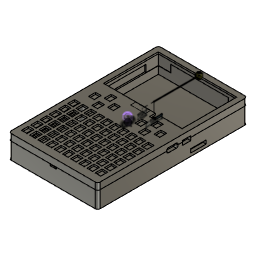
EPI (Autodesk Fusion 360 design; units mm, degrees)
Autodesk Fusion 360 part; units mm, degrees
(part 1 of 2)
sketch "Esquisse1" plane through (0, 0, 0) normal (0, 0, 1) x (1, 0, 0)
  line L0 (33.05, -57.68) -> (-33.05, -57.68)
  line L1 (-33.05, -57.68) -> (-33.05, 57.68)
  line L2 (-33.05, 57.68) -> (33.05, 57.68)
  line L3 (33.05, 57.68) -> (33.05, -57.68)
  line L4 (33.05, -57.68) -> (-33.05, 57.68) construction
  line L5 (-33.05, -57.68) -> (33.05, 57.68) construction
  line L6 (0, 57.68) -> (0, -57.68) construction
  line L7 (31.85, 12.08) -> (-31.85, 12.08)
  line L8 (-31.85, 12.08) -> (-31.85, 56.38)
  line L9 (-31.85, 56.38) -> (31.85, 56.38)
  line L10 (31.85, 56.38) -> (31.85, 12.08)
  line L11 (31.85, 12.08) -> (-31.85, 56.38) construction
  line L12 (-31.85, 12.08) -> (31.85, 56.38) construction
  line L13 (0, -57.68) -> (0, -51.48) construction
  line L14 (0, -51.48) -> (-3.325, -51.48) construction
  line L15 (-1.075, -48.68) -> (-5.575, -48.68)
  line L16 (-5.575, -48.68) -> (-5.575, -54.28)
  line L17 (-5.575, -54.28) -> (-1.075, -54.28)
  line L18 (-1.075, -54.28) -> (-1.075, -48.68)
  line L19 (-1.075, -48.68) -> (-5.575, -54.28) construction
  line L20 (-5.575, -48.68) -> (-1.075, -54.28) construction
  line L21 (-27.675, -48.68) -> (-32.175, -48.68)
  line L22 (-32.175, -48.68) -> (-32.175, -54.28)
  line L23 (-32.175, -54.28) -> (-27.675, -54.28)
  line L24 (-27.675, -54.28) -> (-27.675, -48.68)
  line L25 (-21.025, -48.68) -> (-25.525, -48.68)
  line L26 (-25.525, -48.68) -> (-25.525, -54.28)
  line L27 (-25.525, -54.28) -> (-21.025, -54.28)
  line L28 (-21.025, -54.28) -> (-21.025, -48.68)
  line L29 (-14.375, -48.68) -> (-18.875, -48.68)
  line L30 (-18.875, -48.68) -> (-18.875, -54.28)
  line L31 (-18.875, -54.28) -> (-14.375, -54.28)
  line L32 (-14.375, -54.28) -> (-14.375, -48.68)
  line L33 (-7.725, -48.68) -> (-12.225, -48.68)
  line L34 (-12.225, -48.68) -> (-12.225, -54.28)
  line L35 (-12.225, -54.28) -> (-7.725, -54.28)
  line L36 (-7.725, -54.28) -> (-7.725, -48.68)
  line L37 (5.575, -48.68) -> (1.075, -48.68)
  line L38 (1.075, -48.68) -> (1.075, -54.28)
  line L39 (1.075, -54.28) -> (5.575, -54.28)
  line L40 (5.575, -54.28) -> (5.575, -48.68)
  line L41 (12.225, -48.68) -> (7.725, -48.68)
  line L42 (7.725, -48.68) -> (7.725, -54.28)
  line L43 (7.725, -54.28) -> (12.225, -54.28)
  line L44 (12.225, -54.28) -> (12.225, -48.68)
  line L45 (18.875, -48.68) -> (14.375, -48.68)
  line L46 (14.375, -48.68) -> (14.375, -54.28)
  line L47 (14.375, -54.28) -> (18.875, -54.28)
  line L48 (18.875, -54.28) -> (18.875, -48.68)
  line L49 (25.525, -48.68) -> (21.025, -48.68)
  line L50 (21.025, -48.68) -> (21.025, -54.28)
  line L51 (21.025, -54.28) -> (25.525, -54.28)
  line L52 (25.525, -54.28) -> (25.525, -48.68)
  line L53 (32.175, -48.68) -> (27.675, -48.68)
  line L54 (27.675, -48.68) -> (27.675, -54.28)
  line L55 (27.675, -54.28) -> (32.175, -54.28)
  line L56 (32.175, -54.28) -> (32.175, -48.68)
  line L57 (-27.675, -41.17) -> (-32.175, -41.17)
  line L58 (-32.175, -41.17) -> (-32.175, -46.77)
  line L59 (-32.175, -46.77) -> (-27.675, -46.77)
  line L60 (-27.675, -46.77) -> (-27.675, -41.17)
  line L61 (-21.025, -41.17) -> (-25.525, -41.17)
  line L62 (-25.525, -41.17) -> (-25.525, -46.77)
  line L63 (-25.525, -46.77) -> (-21.025, -46.77)
  line L64 (-21.025, -46.77) -> (-21.025, -41.17)
  line L65 (-14.375, -41.17) -> (-18.875, -41.17)
  line L66 (-18.875, -41.17) -> (-18.875, -46.77)
  line L67 (-18.875, -46.77) -> (-14.375, -46.77)
  line L68 (-14.375, -46.77) -> (-14.375, -41.17)
  line L69 (-7.725, -41.17) -> (-12.225, -41.17)
  line L70 (-12.225, -41.17) -> (-12.225, -46.77)
  line L71 (-12.225, -46.77) -> (-7.725, -46.77)
  line L72 (-7.725, -46.77) -> (-7.725, -41.17)
  line L73 (-1.075, -41.17) -> (-5.575, -41.17)
  line L74 (-5.575, -41.17) -> (-5.575, -46.77)
  line L75 (-5.575, -46.77) -> (-1.075, -46.77)
  line L76 (-1.075, -46.77) -> (-1.075, -41.17)
  line L77 (5.575, -41.17) -> (1.075, -41.17)
  line L78 (1.075, -41.17) -> (1.075, -46.77)
  line L79 (1.075, -46.77) -> (5.575, -46.77)
  line L80 (5.575, -46.77) -> (5.575, -41.17)
  line L81 (12.225, -41.17) -> (7.725, -41.17)
  line L82 (7.725, -41.17) -> (7.725, -46.77)
  line L83 (7.725, -46.77) -> (12.225, -46.77)
  line L84 (12.225, -46.77) -> (12.225, -41.17)
  line L85 (18.875, -41.17) -> (14.375, -41.17)
  line L86 (14.375, -41.17) -> (14.375, -46.77)
  line L87 (14.375, -46.77) -> (18.875, -46.77)
  line L88 (18.875, -46.77) -> (18.875, -41.17)
  line L89 (25.525, -41.17) -> (21.025, -41.17)
  line L90 (21.025, -41.17) -> (21.025, -46.77)
  line L91 (21.025, -46.77) -> (25.525, -46.77)
  line L92 (25.525, -46.77) -> (25.525, -41.17)
  line L93 (32.175, -41.17) -> (27.675, -41.17)
  line L94 (27.675, -41.17) -> (27.675, -46.77)
  line L95 (27.675, -46.77) -> (32.175, -46.77)
  line L96 (32.175, -46.77) -> (32.175, -41.17)
  line L97 (-27.675, -33.66) -> (-32.175, -33.66)
  line L98 (-32.175, -33.66) -> (-32.175, -39.26)
  line L99 (-32.175, -39.26) -> (-27.675, -39.26)
  line L100 (-27.675, -39.26) -> (-27.675, -33.66)
  line L101 (-21.025, -33.66) -> (-25.525, -33.66)
  line L102 (-25.525, -33.66) -> (-25.525, -39.26)
  line L103 (-25.525, -39.26) -> (-21.025, -39.26)
  line L104 (-21.025, -39.26) -> (-21.025, -33.66)
  line L105 (-14.375, -33.66) -> (-18.875, -33.66)
  line L106 (-18.875, -33.66) -> (-18.875, -39.26)
  line L107 (-18.875, -39.26) -> (-14.375, -39.26)
  line L108 (-14.375, -39.26) -> (-14.375, -33.66)
  line L109 (-7.725, -33.66) -> (-12.225, -33.66)
  line L110 (-12.225, -33.66) -> (-12.225, -39.26)
  line L111 (-12.225, -39.26) -> (-7.725, -39.26)
  line L112 (-7.725, -39.26) -> (-7.725, -33.66)
  line L113 (-1.075, -33.66) -> (-5.575, -33.66)
  line L114 (-5.575, -33.66) -> (-5.575, -39.26)
  line L115 (-5.575, -39.26) -> (-1.075, -39.26)
  line L116 (-1.075, -39.26) -> (-1.075, -33.66)
  line L117 (5.575, -33.66) -> (1.075, -33.66)
  line L118 (1.075, -33.66) -> (1.075, -39.26)
  line L119 (1.075, -39.26) -> (5.575, -39.26)
  line L120 (5.575, -39.26) -> (5.575, -33.66)
  line L121 (12.225, -33.66) -> (7.725, -33.66)
  line L122 (7.725, -33.66) -> (7.725, -39.26)
  line L123 (7.725, -39.26) -> (12.225, -39.26)
  line L124 (12.225, -39.26) -> (12.225, -33.66)
  line L125 (18.875, -33.66) -> (14.375, -33.66)
  line L126 (14.375, -33.66) -> (14.375, -39.26)
  line L127 (14.375, -39.26) -> (18.875, -39.26)
  line L128 (18.875, -39.26) -> (18.875, -33.66)
  line L129 (25.525, -33.66) -> (21.025, -33.66)
  line L130 (21.025, -33.66) -> (21.025, -39.26)
  line L131 (21.025, -39.26) -> (25.525, -39.26)
  line L132 (25.525, -39.26) -> (25.525, -33.66)
  line L133 (32.175, -33.66) -> (27.675, -33.66)
  line L134 (27.675, -33.66) -> (27.675, -39.26)
  line L135 (27.675, -39.26) -> (32.175, -39.26)
  line L136 (32.175, -39.26) -> (32.175, -33.66)
  line L137 (-27.675, -26.15) -> (-32.175, -26.15)
  line L138 (-32.175, -26.15) -> (-32.175, -31.75)
  line L139 (-32.175, -31.75) -> (-27.675, -31.75)
  line L140 (-27.675, -31.75) -> (-27.675, -26.15)
  line L141 (-21.025, -26.15) -> (-25.525, -26.15)
  line L142 (-25.525, -26.15) -> (-25.525, -31.75)
  line L143 (-25.525, -31.75) -> (-21.025, -31.75)
  line L144 (-21.025, -31.75) -> (-21.025, -26.15)
  line L145 (-14.375, -26.15) -> (-18.875, -26.15)
  line L146 (-18.875, -26.15) -> (-18.875, -31.75)
  line L147 (-18.875, -31.75) -> (-14.375, -31.75)
  line L148 (-14.375, -31.75) -> (-14.375, -26.15)
  line L149 (-7.725, -26.15) -> (-12.225, -26.15)
  line L150 (-12.225, -26.15) -> (-12.225, -31.75)
  line L151 (-12.225, -31.75) -> (-7.725, -31.75)
  line L152 (-7.725, -31.75) -> (-7.725, -26.15)
  line L153 (-1.075, -26.15) -> (-5.575, -26.15)
  line L154 (-5.575, -26.15) -> (-5.575, -31.75)
  line L155 (-5.575, -31.75) -> (-1.075, -31.75)
  line L156 (-1.075, -31.75) -> (-1.075, -26.15)
  line L157 (5.575, -26.15) -> (1.075, -26.15)
  line L158 (1.075, -26.15) -> (1.075, -31.75)
  line L159 (1.075, -31.75) -> (5.575, -31.75)
  line L160 (5.575, -31.75) -> (5.575, -26.15)
  line L161 (12.225, -26.15) -> (7.725, -26.15)
  line L162 (7.725, -26.15) -> (7.725, -31.75)
  line L163 (7.725, -31.75) -> (12.225, -31.75)
  line L164 (12.225, -31.75) -> (12.225, -26.15)
  line L165 (18.875, -26.15) -> (14.375, -26.15)
  line L166 (14.375, -26.15) -> (14.375, -31.75)
  line L167 (14.375, -31.75) -> (18.875, -31.75)
  line L168 (18.875, -31.75) -> (18.875, -26.15)
  line L169 (25.525, -26.15) -> (21.025, -26.15)
  line L170 (21.025, -26.15) -> (21.025, -31.75)
  line L171 (21.025, -31.75) -> (25.525, -31.75)
  line L172 (25.525, -31.75) -> (25.525, -26.15)
  line L173 (32.175, -26.15) -> (27.675, -26.15)
  line L174 (27.675, -26.15) -> (27.675, -31.75)
  line L175 (27.675, -31.75) -> (32.175, -31.75)
  line L176 (32.175, -31.75) -> (32.175, -26.15)
  line L177 (-27.675, -18.64) -> (-32.175, -18.64)
  line L178 (-32.175, -18.64) -> (-32.175, -24.24)
  line L179 (-32.175, -24.24) -> (-27.675, -24.24)
  line L180 (-27.675, -24.24) -> (-27.675, -18.64)
  line L181 (-21.025, -18.64) -> (-25.525, -18.64)
  line L182 (-25.525, -18.64) -> (-25.525, -24.24)
  line L183 (-25.525, -24.24) -> (-21.025, -24.24)
  line L184 (-21.025, -24.24) -> (-21.025, -18.64)
  line L185 (-14.375, -18.64) -> (-18.875, -18.64)
  line L186 (-18.875, -18.64) -> (-18.875, -24.24)
  line L187 (-18.875, -24.24) -> (-14.375, -24.24)
  line L188 (-14.375, -24.24) -> (-14.375, -18.64)
  line L189 (-7.725, -18.64) -> (-12.225, -18.64)
  line L190 (-12.225, -18.64) -> (-12.225, -24.24)
  line L191 (-12.225, -24.24) -> (-7.725, -24.24)
  line L192 (-7.725, -24.24) -> (-7.725, -18.64)
  line L193 (-1.075, -18.64) -> (-5.575, -18.64)
  line L194 (-5.575, -18.64) -> (-5.575, -24.24)
  line L195 (-5.575, -24.24) -> (-1.075, -24.24)
  line L196 (-1.075, -24.24) -> (-1.075, -18.64)
  line L197 (5.575, -18.64) -> (1.075, -18.64)
  line L198 (1.075, -18.64) -> (1.075, -24.24)
  line L199 (1.075, -24.24) -> (5.575, -24.24)
  line L200 (5.575, -24.24) -> (5.575, -18.64)
  line L201 (12.225, -18.64) -> (7.725, -18.64)
  line L202 (7.725, -18.64) -> (7.725, -24.24)
  line L203 (7.725, -24.24) -> (12.225, -24.24)
  line L204 (12.225, -24.24) -> (12.225, -18.64)
  line L205 (18.875, -18.64) -> (14.375, -18.64)
  line L206 (14.375, -18.64) -> (14.375, -24.24)
  line L207 (14.375, -24.24) -> (18.875, -24.24)
  line L208 (18.875, -24.24) -> (18.875, -18.64)
  line L209 (25.525, -18.64) -> (21.025, -18.64)
  line L210 (21.025, -18.64) -> (21.025, -24.24)
  line L211 (21.025, -24.24) -> (25.525, -24.24)
  line L212 (25.525, -24.24) -> (25.525, -18.64)
  line L213 (32.175, -18.64) -> (27.675, -18.64)
  line L214 (27.675, -18.64) -> (27.675, -24.24)
  line L215 (27.675, -24.24) -> (32.175, -24.24)
  line L216 (32.175, -24.24) -> (32.175, -18.64)
  line L217 (-27.675, -11.13) -> (-32.175, -11.13)
  line L218 (-32.175, -11.13) -> (-32.175, -16.73)
  line L219 (-32.175, -16.73) -> (-27.675, -16.73)
  line L220 (-27.675, -16.73) -> (-27.675, -11.13)
  line L221 (-21.025, -11.13) -> (-25.525, -11.13)
  line L222 (-25.525, -11.13) -> (-25.525, -16.73)
  line L223 (-25.525, -16.73) -> (-21.025, -16.73)
  line L224 (-21.025, -16.73) -> (-21.025, -11.13)
  line L225 (-14.375, -11.13) -> (-18.875, -11.13)
  line L226 (-18.875, -11.13) -> (-18.875, -16.73)
  line L227 (-18.875, -16.73) -> (-14.375, -16.73)
  line L228 (-14.375, -16.73) -> (-14.375, -11.13)
  line L229 (-7.725, -11.13) -> (-12.225, -11.13)
  line L230 (-12.225, -11.13) -> (-12.225, -16.73)
  line L231 (-12.225, -16.73) -> (-7.725, -16.73)
  line L232 (-7.725, -16.73) -> (-7.725, -11.13)
  line L233 (-1.075, -11.13) -> (-5.575, -11.13)
  line L234 (-5.575, -11.13) -> (-5.575, -16.73)
  line L235 (-5.575, -16.73) -> (-1.075, -16.73)
  line L236 (-1.075, -16.73) -> (-1.075, -11.13)
  line L237 (5.575, -11.13) -> (1.075, -11.13)
  line L238 (1.075, -11.13) -> (1.075, -16.73)
  line L239 (1.075, -16.73) -> (5.575, -16.73)
  line L240 (5.575, -16.73) -> (5.575, -11.13)
  line L241 (12.225, -11.13) -> (7.725, -11.13)
  line L242 (7.725, -11.13) -> (7.725, -16.73)
  line L243 (7.725, -16.73) -> (12.225, -16.73)
  line L244 (12.225, -16.73) -> (12.225, -11.13)
  line L245 (18.875, -11.13) -> (14.375, -11.13)
  line L246 (14.375, -11.13) -> (14.375, -16.73)
  line L247 (14.375, -16.73) -> (18.875, -16.73)
  line L248 (18.875, -16.73) -> (18.875, -11.13)
  line L249 (25.525, -11.13) -> (21.025, -11.13)
  line L250 (21.025, -11.13) -> (21.025, -16.73)
  line L251 (21.025, -16.73) -> (25.525, -16.73)
  line L252 (25.525, -16.73) -> (25.525, -11.13)
  line L253 (32.175, -11.13) -> (27.675, -11.13)
  line L254 (27.675, -11.13) -> (27.675, -16.73)
  line L255 (27.675, -16.73) -> (32.175, -16.73)
  line L256 (32.175, -16.73) -> (32.175, -11.13)
  line L257 (-5.8196, -10.1565) -> (33.05, -10.1565)
  line L258 (33.05, 57.68) -> (33.05, -0.32) construction
  line L259 (33.05, -0.32) -> (26.57, -0.32) construction
  line L260 (26.57, -0.32) -> (11.1, -0.32) construction
  line L261 (13.35, -3.12) -> (8.85, -3.12)
  line L262 (8.85, -3.12) -> (8.85, 2.48)
  line L263 (8.85, 2.48) -> (13.35, 2.48)
  line L264 (13.35, 2.48) -> (13.35, -3.12)
  line L265 (13.35, -3.12) -> (8.85, 2.48) construction
  line L266 (8.85, -3.12) -> (13.35, 2.48) construction
  line L267 (28.82, -3.12) -> (24.32, -3.12)
  line L268 (24.32, -3.12) -> (24.32, 2.48)
  line L269 (24.32, 2.48) -> (28.82, 2.48)
  line L270 (28.82, 2.48) -> (28.82, -3.12)
  line L271 (28.82, -3.12) -> (24.32, 2.48) construction
  line L272 (24.32, -3.12) -> (28.82, 2.48) construction
  line L273 (18.835, -0.32) -> (18.835, 4.71) construction
  line L274 (18.835, -0.32) -> (18.835, -5.35) construction
  line L275 (21.085, 1.91) -> (16.585, 1.91)
  line L276 (16.585, 1.91) -> (16.585, 7.51)
  line L277 (16.585, 7.51) -> (21.085, 7.51)
  line L278 (21.085, 7.51) -> (21.085, 1.91)
  line L279 (21.085, 1.91) -> (16.585, 7.51) construction
  line L280 (16.585, 1.91) -> (21.085, 7.51) construction
  line L281 (21.085, -8.15) -> (16.585, -8.15)
  line L282 (16.585, -8.15) -> (16.585, -2.55)
  line L283 (16.585, -2.55) -> (21.085, -2.55)
  line L284 (21.085, -2.55) -> (21.085, -8.15)
  line L285 (21.085, -8.15) -> (16.585, -2.55) construction
  line L286 (16.585, -8.15) -> (21.085, -2.55) construction
  line L287 (-21.085, 1.91) -> (-16.585, 1.91)
  line L288 (-21.085, 7.51) -> (-21.085, 1.91)
  line L289 (-16.585, 7.51) -> (-21.085, 7.51)
  line L290 (-16.585, 1.91) -> (-16.585, 7.51)
  line L291 (-21.085, -2.55) -> (-21.085, -8.15)
  line L292 (-16.585, -2.55) -> (-21.085, -2.55)
  line L293 (-16.585, -8.15) -> (-16.585, -2.55)
  line L294 (-21.085, -8.15) -> (-16.585, -8.15)
  line L295 (-24.32, -3.12) -> (-24.32, 2.48)
  line L296 (-24.32, 2.48) -> (-28.82, 2.48)
  line L297 (-28.82, 2.48) -> (-28.82, -3.12)
  line L298 (-28.82, -3.12) -> (-24.32, -3.12)
  line L299 (-8.85, -3.12) -> (-8.85, 2.48)
  line L300 (-8.85, 2.48) -> (-13.35, 2.48)
  line L301 (-13.35, 2.48) -> (-13.35, -3.12)
  line L302 (-13.35, -3.12) -> (-8.85, -3.12)
  line L303 (33.05, 57.68) -> (33.05, 10.18) construction
  line L304 (33.05, 10.18) -> (12.35, 10.18) construction
  line L305 (14.6, 7.38) -> (10.1, 7.38)
  line L306 (10.1, 7.38) -> (10.1, 12.98)
  line L307 (10.1, 12.98) -> (14.6, 12.98)
  line L308 (14.6, 12.98) -> (14.6, 7.38)
  line L309 (14.6, 7.38) -> (10.1, 12.98) construction
  line L310 (10.1, 7.38) -> (14.6, 12.98) construction
  line L311 (0, 12.08) -> (6, 12.08)
  line L312 (6, 12.08) -> (6, 8.08)
  line L313 (6, 8.08) -> (0, 8.08)
  line L314 (0, 8.08) -> (0, 12.08)
  line L315 (0, 12.08) -> (-6, 12.08)
  line L316 (-6, 12.08) -> (-6, 8.08)
  line L317 (-6, 8.08) -> (0, 8.08)
  line L318 (0, 8.08) -> (0, 12.08)
  line L319 (33.45, 58.08) -> (33.45, -58.08)
  line L320 (33.45, -58.08) -> (-33.45, -58.08)
  line L321 (-33.45, -58.08) -> (-33.45, 58.08)
  line L322 (-33.45, 58.08) -> (33.45, 58.08)
  line L323 (36.05, 58.68) -> (36.05, -58.68)
  line L324 (34.05, -60.68) -> (-34.05, -60.68)
  line L325 (-36.05, -58.68) -> (-36.05, 58.68)
  line L326 (-34.05, 60.68) -> (34.05, 60.68)
  arc A0 (-34.05, 60.68) -> (-36.05, 58.68) centre (-34.05, 58.68) ccw
  arc A1 (36.05, 58.68) -> (34.05, 60.68) centre (34.05, 58.68) ccw
  arc A2 (34.05, -60.68) -> (36.05, -58.68) centre (34.05, -58.68) ccw
  arc A3 (-36.05, -58.68) -> (-34.05, -60.68) centre (-34.05, -58.68) ccw
  line L327 (33.45, 58.08) -> (23.45, 58.08)
  line L328 (33.45, 58.08) -> (33.45, 48.08)
  line L329 (33.45, 48.08) -> (34.45, 48.08)
  line L330 (23.45, 58.08) -> (23.45, 59.08)
  line L331 (34.45, 48.08) -> (34.45, 59.08)
  line L332 (23.45, 59.08) -> (34.45, 59.08)
  line L333 (33.45, -58.08) -> (23.45, -58.08)
  line L334 (33.45, -58.08) -> (33.45, -48.08)
  line L335 (33.45, -48.08) -> (34.45, -48.08)
  line L336 (23.45, -58.08) -> (23.45, -59.08)
  line L337 (34.45, -48.08) -> (34.45, -59.08)
  line L338 (23.45, -59.08) -> (34.45, -59.08)
  line L339 (34.65, -47.88) -> (34.65, -59.28)
  line L340 (23.25, -59.28) -> (34.65, -59.28)
  line L341 (23.25, -57.88) -> (23.25, -59.28)
  line L342 (33.25, -57.88) -> (23.25, -57.88)
  line L343 (33.25, -57.88) -> (33.25, -47.88)
  line L344 (33.25, -47.88) -> (34.65, -47.88)
  line L345 (23.25, 59.28) -> (34.65, 59.28)
  line L346 (34.65, 47.88) -> (34.65, 59.28)
  line L347 (33.25, 47.88) -> (34.65, 47.88)
  line L348 (33.25, 57.88) -> (33.25, 47.88)
  line L349 (33.25, 57.88) -> (23.25, 57.88)
  line L350 (23.25, 57.88) -> (23.25, 59.28)
  line L351 (-34.45, 48.08) -> (-34.45, 59.08)
  line L352 (-23.45, 59.08) -> (-34.45, 59.08)
  line L353 (-23.25, 59.28) -> (-34.65, 59.28)
  line L354 (-34.65, 47.88) -> (-34.65, 59.28)
  line L355 (-33.25, 47.88) -> (-34.65, 47.88)
  line L356 (-33.45, 48.08) -> (-34.45, 48.08)
  line L357 (-23.25, 57.88) -> (-23.25, 59.28)
  line L358 (-23.45, 58.08) -> (-23.45, 59.08)
  line L359 (-34.45, -48.08) -> (-34.45, -59.08)
  line L360 (-34.65, -47.88) -> (-34.65, -59.28)
  line L361 (-33.25, -47.88) -> (-34.65, -47.88)
  line L362 (-33.45, -48.08) -> (-34.45, -48.08)
  line L363 (-23.25, -59.28) -> (-34.65, -59.28)
  line L364 (-23.45, -59.08) -> (-34.45, -59.08)
  line L365 (-23.25, -57.88) -> (-23.25, -59.28)
  line L366 (-23.45, -58.08) -> (-23.45, -59.08)
  line L367 (-34.65, -47.88) -> (-34.65, 47.88)
  point P0 (0, 34.23)
  point P1 (-3.325, -51.48)
  point P2 (11.1, -0.32)
  point P3 (26.57, -0.32)
  point P4 (18.835, 4.71)
  point P5 (18.835, -5.35)
  point P6 (12.35, 10.18)
  dimension "d12" = 66.1
  dimension "d13" = 115.36
  dimension "d14" = 63.7
  dimension "d15" = 44.3
  dimension "d16" = 1.3
  dimension "d20" = 6.2
  dimension "d21" = 3.325
  dimension "d22" = 4.5
  dimension "d23" = 5.6
  dimension "d26" = 6.65
  dimension "d27" = 7.51
  dimension "d33" = 58
  dimension "d34" = 6.48
  dimension "d35" = 15.47
  dimension "d36" = 4.5
  dimension "d37" = 5.6
  dimension "d38" = 4.5
  dimension "d39" = 5.6
  dimension "d40" = 5.03
  dimension "d41" = 5.03
  dimension "d42" = 4.5
  dimension "d43" = 5.6
  dimension "d44" = 4.5
  dimension "d45" = 5.6
  dimension "d46" = 47.5
  dimension "d47" = 20.7
  dimension "d48" = 4.5
  dimension "d49" = 5.6
  dimension "d74" = 6
  dimension "d75" = 4
  dimension "d76" = 6
  dimension "d77" = 4
  dimension "d83" = 2
  dimension "d98" = 10
  dimension "d99" = 10
  dimension "d101" = 1
  dimension "d102" = 1
  dimension "d103" = 11
  dimension "d104" = 11
  dimension "d106" = 10
  dimension "d107" = 10
  dimension "d108" = 1
  dimension "d109" = 1
  dimension "d110" = 11
  dimension "d111" = 11
  constraint horizontal L0
  constraint perpendicular L0 L1
  constraint parallel L0 L2
  constraint parallel L1 L3
  constraint coincident L4 origin
  constraint coincident L5 origin
  constraint midpoint L2 L6.start
  constraint midpoint L0 L6.end
  constraint horizontal L7
  constraint perpendicular L7 L8
  constraint parallel L7 L9
  constraint parallel L8 L10
  constraint coincident L11 P0
  constraint coincident L12 P0
  constraint coincident L6 P0
  constraint perpendicular L0 L13
  constraint perpendicular L3 L14
  constraint horizontal L15
  constraint perpendicular L15 L16
  constraint parallel L15 L17
  constraint parallel L16 L18
  constraint coincident L19 P1
  constraint coincident L20 P1
  constraint coincident P1 L14.end
  constraint coincident L3 L257.end
  constraint perpendicular L3 L257
  constraint perpendicular L7 L258
  constraint perpendicular L258 L259
  constraint perpendicular L6 L260
  constraint horizontal L261
  constraint perpendicular L261 L262
  constraint parallel L261 L263
  constraint parallel L262 L264
  constraint coincident L265 P2
  constraint coincident L266 P2
  constraint coincident P2 L260.end
  constraint horizontal L267
  constraint perpendicular L267 L268
  constraint parallel L267 L269
  constraint parallel L268 L270
  constraint coincident L271 P3
  constraint coincident L272 P3
  constraint coincident P3 L259.end
  constraint midpoint L260 L273.start
  constraint perpendicular L7 L273
  constraint perpendicular L260 L274
  constraint horizontal L275
  constraint perpendicular L275 L276
  constraint parallel L275 L277
  constraint parallel L276 L278
  constraint coincident L279 P4
  constraint coincident L280 P4
  constraint coincident P4 L273.end
  constraint horizontal L281
  constraint perpendicular L281 L282
  constraint parallel L281 L283
  constraint parallel L282 L284
  constraint coincident L285 P5
  constraint coincident L286 P5
  constraint coincident P5 L274.end
  constraint symmetric L6 L261.start L301.end
  constraint symmetric L6 L261.end L299.start
  constraint symmetric L6 L262.end L299.end
  constraint symmetric L6 L263.end L300.end
  constraint symmetric L6 L267.start L297.end
  constraint symmetric L6 L267.end L295.start
  constraint symmetric L6 L268.end L295.end
  constraint symmetric L6 L269.end L296.end
  constraint symmetric L6 L275.start L287.start
  constraint symmetric L6 L275.end L287.end
  constraint symmetric L6 L276.end L289.start
  constraint symmetric L6 L277.end L288.start
  constraint symmetric L6 L281.start L291.end
  constraint symmetric L6 L281.end L293.start
  constraint symmetric L6 L282.end L292.start
  constraint symmetric L6 L283.end L291.start
  constraint perpendicular L2 L303
  constraint perpendicular L303 L304
  constraint horizontal L305
  constraint perpendicular L305 L306
  constraint parallel L305 L307
  constraint parallel L306 L308
  constraint coincident L309 P6
  constraint coincident L310 P6
  constraint coincident P6 L304.end
  constraint coincident L5 L257.start
  constraint horizontal L311
  constraint vertical L312
  constraint horizontal L313
  constraint vertical L314
  constraint midpoint L7 L311.start
  constraint horizontal L315
  constraint vertical L316
  constraint horizontal L317
  constraint vertical L318
  constraint tangent L325 A0
  constraint tangent L326 A0
  constraint tangent L323 A1
  constraint tangent L326 A1
  constraint equal A0 A1
  constraint tangent L323 A2
  constraint tangent L324 A2
  constraint equal A0 A2
  constraint tangent L324 A3
  constraint tangent L325 A3
  constraint equal A0 A3
  constraint coincident L322 L327.end
  constraint coincident L319 L328.end
  constraint perpendicular L328 L329
  constraint perpendicular L327 L330
  constraint perpendicular L329 L331
  constraint perpendicular L330 L332
  constraint perpendicular L319 L333
  constraint perpendicular L320 L334
  constraint perpendicular L334 L335
  constraint perpendicular L333 L336
  constraint perpendicular L335 L337
  constraint perpendicular L336 L338
  constraint symmetric L6 L327.end L358.start
  constraint symmetric L6 L328.end L356.start
  constraint symmetric L6 L329.end L351.start
  constraint symmetric L6 L330.end L352.start
  constraint symmetric L6 L331.end L351.end
  constraint symmetric L6 L333.end L366.start
  constraint symmetric L6 L334.end L362.start
  constraint symmetric L6 L335.end L359.start
  constraint symmetric L6 L336.end L364.start
  constraint symmetric L6 L337.end L359.end
  constraint symmetric L6 L339.start L360.start
  constraint symmetric L6 L339.end L360.end
  constraint symmetric L6 L340.start L363.start
  constraint symmetric L6 L341.start L365.start
  constraint symmetric L6 L343.end L361.start
  constraint symmetric L6 L345.start L353.start
  constraint symmetric L6 L345.end L353.end
  constraint symmetric L6 L346.start L354.start
  constraint symmetric L6 L347.start L355.start
  constraint symmetric L6 L349.end L357.start
  measures "d12" distance of L1.end L2.end
  measures "d13" distance of L0.end L1.end
  measures "d14" distance of L8.end L9.end
  measures "d15" distance of L7.end L8.end
  measures "d16" distance of L2 L9
  measures "d20" distance of L6.end L13.end
  measures "d21" distance of L13.end P1
  measures "d22" distance of L16.end L17.end
  measures "d23" distance of L15.end L16.end
  measures "d33" distance of L2.end L258.end
  measures "d34" distance of L258.end P3
  measures "d35" distance of P3 P2
  measures "d36" distance of L262.end L263.end
  measures "d37" distance of L261.end L262.end
  measures "d38" distance of L268.end L269.end
  measures "d39" distance of L267.end L268.end
  measures "d40" distance of L273.start P4
  measures "d41" distance of L273.start P5
  measures "d42" distance of L276.end L277.end
  measures "d43" distance of L275.end L276.end
  measures "d44" distance of L282.end L283.end
  measures "d45" distance of L281.end L282.end
  measures "d46" distance of L2.end L303.end
  measures "d47" distance of L303.end P6
  measures "d48" distance of L306.end L307.end
  measures "d49" distance of L305.end L306.end
  measures "d74" distance of L311.start L311.end
  measures "d75" distance of L311.start L313.end
  measures "d76" distance of L311.start L315.end
  measures "d77" distance of L311.start L313.end
  measures "d83" radius of A0
  measures "d98" distance of L319.start L327.end
  measures "d99" distance of L319.start L328.end
  measures "d101" distance of L328.end L329.end
  measures "d102" distance of L327.end L330.end
  measures "d103" distance of L329.end L331.end
  measures "d104" distance of L330.end L331.end
  measures "d106" distance of L319.end L333.end
  measures "d107" distance of L319.end L334.end
  measures "d108" distance of L334.end L335.end
  measures "d109" distance of L333.end L336.end
  measures "d110" distance of L335.end L337.end
  measures "d111" distance of L336.end L337.end
sketch "Esquisse2" plane through (0, 0, 0) normal (1, 0, 0) x (0, 1, 0)
  line L0 (0, 0) -> (0, -4) construction
  line L1 (3.15, -2.2) -> (-3.15, -2.2)
  line L2 (-4.65, -3.7) -> (-4.65, -4.3)
  line L3 (-3.15, -5.8) -> (3.15, -5.8)
  line L4 (4.65, -4.3) -> (4.65, -3.7)
  line L5 (4.65, -2.2) -> (-4.65, -5.8) construction
  line L6 (-4.65, -2.2) -> (4.65, -5.8) construction
  arc A0 (-3.15, -2.2) -> (-4.65, -3.7) centre (-3.15, -3.7) ccw
  arc A1 (-4.65, -4.3) -> (-3.15, -5.8) centre (-3.15, -4.3) ccw
  arc A2 (4.65, -3.7) -> (3.15, -2.2) centre (3.15, -3.7) ccw
  arc A3 (3.15, -5.8) -> (4.65, -4.3) centre (3.15, -4.3) ccw
  line L7 (57.68, 0) -> (11.56, 0) construction
  line L8 (11.56, 0) -> (11.56, -4.58) construction
  line L9 (14.91, -2.83) -> (8.21, -2.83)
  line L10 (8.21, -2.83) -> (8.21, -6.33)
  line L11 (8.21, -6.33) -> (14.91, -6.33)
  line L12 (14.91, -6.33) -> (14.91, -2.83)
  line L13 (14.91, -2.83) -> (8.21, -6.33) construction
  line L14 (8.21, -2.83) -> (14.91, -6.33) construction
  line L15 (57.68, 0) -> (21.08, 0)
  line L16 (21.08, 0) -> (21.08, -13.5) construction
  line L17 (27.38, -15) -> (14.78, -15)
  line L18 (14.78, -15) -> (14.78, -12)
  line L19 (14.78, -12) -> (27.38, -12)
  line L20 (27.38, -12) -> (27.38, -15)
  line L21 (27.38, -15) -> (14.78, -12) construction
  line L22 (14.78, -15) -> (27.38, -12) construction
  point P0 (-0.32, 0)
  point P1 (0, -4)
  point P2 (57.68, 0)
  point P3 (11.56, -4.58)
  point P4 (21.08, -13.5)
  dimension "d60" = 4
  dimension "d63" = 9.3
  dimension "d64" = 3.6
  dimension "d65" = 1.5
  dimension "d66" = 46.12
  dimension "d67" = 4.58
  dimension "d70" = 6.7
  dimension "d71" = 3.5
  dimension "d130" = 36.6
  dimension "d131" = 13.5
  dimension "d132" = 12.6
  dimension "d133" = 3
  constraint coincident L0.start origin
  constraint vertical L0
  constraint horizontal L1
  constraint perpendicular L1 L2
  constraint parallel L1 L3
  constraint parallel L2 L4
  constraint coincident L5 P1
  constraint coincident L6 P1
  constraint coincident P1 L0.end
  constraint coincident L6.start L2
  constraint coincident L6.start L1
  constraint tangent L2 A0
  constraint tangent L1 A0
  constraint coincident L5.end L3
  constraint coincident L5.end L2
  constraint tangent L3 A1
  constraint tangent L2 A1
  constraint equal A0 A1
  constraint coincident L5.start L1
  constraint coincident L5.start L4
  constraint tangent L1 A2
  constraint tangent L4 A2
  constraint equal A0 A2
  constraint coincident L6.end L3
  constraint coincident L6.end L4
  constraint tangent L3 A3
  constraint tangent L4 A3
  constraint equal A0 A3
  constraint coincident P2 L7.start
  constraint horizontal L7
  constraint perpendicular L3 L8
  constraint horizontal L9
  constraint perpendicular L9 L10
  constraint parallel L9 L11
  constraint parallel L10 L12
  constraint coincident L13 P3
  constraint coincident L14 P3
  constraint coincident P3 L8.end
  constraint parallel L7 L15
  constraint perpendicular L15 L16
  constraint horizontal L17
  constraint perpendicular L17 L18
  constraint parallel L17 L19
  constraint parallel L18 L20
  constraint coincident L21 P4
  constraint coincident L22 P4
  constraint coincident P4 L16.end
  measures "d60" distance of L0.start P1
  measures "d63" distance of L5.end L6.end
  measures "d64" distance of L6.start L5.end
  measures "d65" radius of A0
  measures "d66" distance of P2 L7.end
  measures "d67" distance of L7.end P3
  measures "d70" distance of L10.end L11.end
  measures "d71" distance of L9.end L10.end
  measures "d130" distance of P2 L15.end
  measures "d131" distance of L15.end P4
  measures "d132" distance of L18.end L19.end
  measures "d133" distance of L17.end L18.end
extrude "Extrusion7" add sketch "Esquisse1" along normal blind 1.4 contours L0 L1 L2 L3 | L7 L311 L312 L313 L314 L318 | L7 L314 L315 L316 L317 L318 | L319 L322 L327 L328 L329 L330 L331 L332 | L319 L322 L327 L328 L347 L348 L349 L350 | L319 L322 L329 L330 L331 L332 L345 L346 L347 L350 | L319 L320 L321 L322 L341 L342 L343 L344 L347 L348 L349 L350 | L319 L320 L335 L336 L337 L338 L339 L340 L341 L344 | L319 L320 L333 L334 L341 L342 L343 L344 | L321 L322 L351 L352 L353 L354 L355 L356 L357 L358 | L319 L320 L333 L334 L335 L336 L337 L338 | L321 L322 L351 L352 L356 L358 | L321 L355 L361 L367 | L320 L321 L359 L360 L361 L362 L363 L364 L365 L366 | L320 L321 L359 L362 L364 L366 | L323 L324 L325 L326 A0 A1 A2 A3 makes body 1
extrude "Extrusion8" add sketch "Esquisse1" against normal blind 4 contours L319 L322 L327 L328 L329 L330 L331 L332 | L319 L322 L329 L330 L331 L332 L345 L346 L347 L350 | L319 L320 L335 L336 L337 L338 L339 L340 L341 L344 | L321 L322 L351 L352 L353 L354 L355 L356 L357 L358 | L319 L320 L333 L334 L335 L336 L337 L338 | L321 L322 L351 L352 L356 L358 | L321 L355 L361 L367 | L320 L321 L359 L360 L361 L362 L363 L364 L365 L366 | L320 L321 L359 L362 L364 L366 | L323 L324 L325 L326 A0 A1 A2 A3 bodies 1
extrude "Extrusion9" cut sketch "Esquisse1" along normal blind 1 contours L7 L311 L312 L313 L314 L318 | L7 L314 L315 L316 L317 L318 bodies 1
ref_plane "Plan de construction1" through (0, 0, -16) normal (0, 0, 1) x (1, 0, 0)
sketch "Esquisse3" plane through (0, 0, -16) normal (0, 0, 1) x (1, 0, 0)
  line L0 (-33.45, 58.08) -> (-33.45, -58.08)
  line L1 (-33.45, -58.08) -> (33.45, -58.08)
  line L2 (33.45, -58.08) -> (33.45, 58.08)
  line L3 (33.45, 58.08) -> (-33.45, 58.08)
  arc A0 (-34.05, 60.68) -> (-36.05, 58.68) centre (-33.45, 58.08) ccw
  line L4 (-34.05, 60.68) -> (34.05, 60.68)
  arc A1 (36.05, 58.68) -> (34.05, 60.68) centre (33.45, 58.08) ccw
  line L5 (36.05, 58.68) -> (36.05, -58.68)
  arc A2 (34.05, -60.68) -> (36.05, -58.68) centre (33.45, -58.08) ccw
  line L6 (34.05, -60.68) -> (-34.05, -60.68)
  arc A3 (-36.05, -58.68) -> (-34.05, -60.68) centre (-33.45, -58.08) ccw
  line L7 (-36.05, -58.68) -> (-36.05, 58.68)
  line L8 (5.575, -11.13) -> (5.575, -16.73)
  line L9 (5.575, -16.73) -> (1.075, -16.73)
  line L10 (1.075, -16.73) -> (1.075, -11.13)
  line L11 (1.075, -11.13) -> (5.575, -11.13)
  line L12 (18.875, -18.64) -> (18.875, -24.24)
  line L13 (18.875, -24.24) -> (14.375, -24.24)
  line L14 (14.375, -24.24) -> (14.375, -18.64)
  line L15 (14.375, -18.64) -> (18.875, -18.64)
  line L16 (5.575, -18.64) -> (5.575, -24.24)
  line L17 (5.575, -24.24) -> (1.075, -24.24)
  line L18 (1.075, -24.24) -> (1.075, -18.64)
  line L19 (1.075, -18.64) -> (5.575, -18.64)
  line L20 (-1.075, -18.64) -> (-1.075, -24.24)
  line L21 (-1.075, -24.24) -> (-5.575, -24.24)
  line L22 (-5.575, -24.24) -> (-5.575, -18.64)
  line L23 (-5.575, -18.64) -> (-1.075, -18.64)
  line L24 (-7.725, -18.64) -> (-7.725, -24.24)
  line L25 (-7.725, -24.24) -> (-12.225, -24.24)
  line L26 (-12.225, -24.24) -> (-12.225, -18.64)
  line L27 (-12.225, -18.64) -> (-7.725, -18.64)
  line L28 (-14.375, -18.64) -> (-14.375, -24.24)
  line L29 (-14.375, -24.24) -> (-18.875, -24.24)
  line L30 (-18.875, -24.24) -> (-18.875, -18.64)
  line L31 (-18.875, -18.64) -> (-14.375, -18.64)
  line L32 (-21.025, -18.64) -> (-21.025, -24.24)
  line L33 (-21.025, -24.24) -> (-25.525, -24.24)
  line L34 (-25.525, -24.24) -> (-25.525, -18.64)
  line L35 (-25.525, -18.64) -> (-21.025, -18.64)
  line L36 (-27.675, -18.64) -> (-27.675, -24.24)
  line L37 (-27.675, -24.24) -> (-32.175, -24.24)
  line L38 (-32.175, -24.24) -> (-32.175, -18.64)
  line L39 (-32.175, -18.64) -> (-27.675, -18.64)
  line L40 (32.175, -26.15) -> (32.175, -31.75)
  line L41 (32.175, -31.75) -> (27.675, -31.75)
  line L42 (27.675, -31.75) -> (27.675, -26.15)
  line L43 (27.675, -26.15) -> (32.175, -26.15)
  line L44 (25.525, -26.15) -> (25.525, -31.75)
  line L45 (25.525, -31.75) -> (21.025, -31.75)
  line L46 (21.025, -31.75) -> (21.025, -26.15)
  line L47 (21.025, -26.15) -> (25.525, -26.15)
  line L48 (18.875, -26.15) -> (18.875, -31.75)
  line L49 (18.875, -31.75) -> (14.375, -31.75)
  line L50 (14.375, -31.75) -> (14.375, -26.15)
  line L51 (14.375, -26.15) -> (18.875, -26.15)
  line L52 (12.225, -26.15) -> (12.225, -31.75)
  line L53 (12.225, -31.75) -> (7.725, -31.75)
  line L54 (7.725, -31.75) -> (7.725, -26.15)
  line L55 (7.725, -26.15) -> (12.225, -26.15)
  line L56 (5.575, -26.15) -> (5.575, -31.75)
  line L57 (5.575, -31.75) -> (1.075, -31.75)
  line L58 (1.075, -31.75) -> (1.075, -26.15)
  line L59 (1.075, -26.15) -> (5.575, -26.15)
  line L60 (-1.075, -26.15) -> (-1.075, -31.75)
  line L61 (-1.075, -31.75) -> (-5.575, -31.75)
  line L62 (-5.575, -31.75) -> (-5.575, -26.15)
  line L63 (-5.575, -26.15) -> (-1.075, -26.15)
  line L64 (-7.725, -26.15) -> (-7.725, -31.75)
  line L65 (-7.725, -31.75) -> (-12.225, -31.75)
  line L66 (-12.225, -31.75) -> (-12.225, -26.15)
  line L67 (-12.225, -26.15) -> (-7.725, -26.15)
  line L68 (-14.375, -26.15) -> (-14.375, -31.75)
  line L69 (-14.375, -31.75) -> (-18.875, -31.75)
  line L70 (-18.875, -31.75) -> (-18.875, -26.15)
  line L71 (-18.875, -26.15) -> (-14.375, -26.15)
  line L72 (-21.025, -26.15) -> (-21.025, -31.75)
  line L73 (-21.025, -31.75) -> (-25.525, -31.75)
  line L74 (-25.525, -31.75) -> (-25.525, -26.15)
  line L75 (-25.525, -26.15) -> (-21.025, -26.15)
  line L76 (-27.675, -26.15) -> (-27.675, -31.75)
  line L77 (-27.675, -31.75) -> (-32.175, -31.75)
  line L78 (-32.175, -31.75) -> (-32.175, -26.15)
  line L79 (-32.175, -26.15) -> (-27.675, -26.15)
  line L80 (25.525, -33.66) -> (25.525, -39.26)
  line L81 (25.525, -39.26) -> (21.025, -39.26)
  line L82 (21.025, -39.26) -> (21.025, -33.66)
  line L83 (21.025, -33.66) -> (25.525, -33.66)
  line L84 (32.175, -33.66) -> (32.175, -39.26)
  line L85 (32.175, -39.26) -> (27.675, -39.26)
  line L86 (27.675, -39.26) -> (27.675, -33.66)
  line L87 (27.675, -33.66) -> (32.175, -33.66)
  line L88 (18.875, -33.66) -> (18.875, -39.26)
  line L89 (18.875, -39.26) -> (14.375, -39.26)
  line L90 (14.375, -39.26) -> (14.375, -33.66)
  line L91 (14.375, -33.66) -> (18.875, -33.66)
  line L92 (12.225, -33.66) -> (12.225, -39.26)
  line L93 (12.225, -39.26) -> (7.725, -39.26)
  line L94 (7.725, -39.26) -> (7.725, -33.66)
  line L95 (7.725, -33.66) -> (12.225, -33.66)
  line L96 (5.575, -33.66) -> (5.575, -39.26)
  line L97 (5.575, -39.26) -> (1.075, -39.26)
  line L98 (1.075, -39.26) -> (1.075, -33.66)
  line L99 (1.075, -33.66) -> (5.575, -33.66)
  line L100 (-7.725, -33.66) -> (-7.725, -39.26)
  line L101 (-7.725, -39.26) -> (-12.225, -39.26)
  line L102 (-12.225, -39.26) -> (-12.225, -33.66)
  line L103 (-12.225, -33.66) -> (-7.725, -33.66)
  line L104 (-1.075, -33.66) -> (-1.075, -39.26)
  line L105 (-1.075, -39.26) -> (-5.575, -39.26)
  line L106 (-5.575, -39.26) -> (-5.575, -33.66)
  line L107 (-5.575, -33.66) -> (-1.075, -33.66)
  line L108 (-14.375, -33.66) -> (-14.375, -39.26)
  line L109 (-14.375, -39.26) -> (-18.875, -39.26)
  line L110 (-18.875, -39.26) -> (-18.875, -33.66)
  line L111 (-18.875, -33.66) -> (-14.375, -33.66)
  line L112 (-21.025, -33.66) -> (-21.025, -39.26)
  line L113 (-21.025, -39.26) -> (-25.525, -39.26)
  line L114 (-25.525, -39.26) -> (-25.525, -33.66)
  line L115 (-25.525, -33.66) -> (-21.025, -33.66)
  line L116 (-1.075, -41.17) -> (-1.075, -46.77)
  line L117 (-1.075, -46.77) -> (-5.575, -46.77)
  line L118 (-5.575, -46.77) -> (-5.575, -41.17)
  line L119 (-5.575, -41.17) -> (-1.075, -41.17)
  line L120 (5.575, -41.17) -> (5.575, -46.77)
  line L121 (5.575, -46.77) -> (1.075, -46.77)
  line L122 (1.075, -46.77) -> (1.075, -41.17)
  line L123 (1.075, -41.17) -> (5.575, -41.17)
  line L124 (12.225, -41.17) -> (12.225, -46.77)
  line L125 (12.225, -46.77) -> (7.725, -46.77)
  line L126 (7.725, -46.77) -> (7.725, -41.17)
  line L127 (7.725, -41.17) -> (12.225, -41.17)
  line L128 (18.875, -41.17) -> (18.875, -46.77)
  line L129 (18.875, -46.77) -> (14.375, -46.77)
  line L130 (14.375, -46.77) -> (14.375, -41.17)
  line L131 (14.375, -41.17) -> (18.875, -41.17)
  line L132 (25.525, -41.17) -> (25.525, -46.77)
  line L133 (25.525, -46.77) -> (21.025, -46.77)
  line L134 (21.025, -46.77) -> (21.025, -41.17)
  line L135 (21.025, -41.17) -> (25.525, -41.17)
  line L136 (-27.675, -33.66) -> (-27.675, -39.26)
  line L137 (-27.675, -39.26) -> (-32.175, -39.26)
  line L138 (-32.175, -39.26) -> (-32.175, -33.66)
  line L139 (-32.175, -33.66) -> (-27.675, -33.66)
  line L140 (32.175, -41.17) -> (32.175, -46.77)
  line L141 (32.175, -46.77) -> (27.675, -46.77)
  line L142 (27.675, -46.77) -> (27.675, -41.17)
  line L143 (27.675, -41.17) -> (32.175, -41.17)
  line L144 (12.225, -18.64) -> (12.225, -24.24)
  line L145 (12.225, -24.24) -> (7.725, -24.24)
  line L146 (7.725, -24.24) -> (7.725, -18.64)
  line L147 (7.725, -18.64) -> (12.225, -18.64)
  line L148 (25.525, -18.64) -> (25.525, -24.24)
  line L149 (25.525, -24.24) -> (21.025, -24.24)
  line L150 (21.025, -24.24) -> (21.025, -18.64)
  line L151 (21.025, -18.64) -> (25.525, -18.64)
  line L152 (32.175, -18.64) -> (32.175, -24.24)
  line L153 (32.175, -24.24) -> (27.675, -24.24)
  line L154 (27.675, -24.24) -> (27.675, -18.64)
  line L155 (27.675, -18.64) -> (32.175, -18.64)
  line L156 (-27.675, -11.13) -> (-27.675, -16.73)
  line L157 (-27.675, -16.73) -> (-32.175, -16.73)
  line L158 (-32.175, -16.73) -> (-32.175, -11.13)
  line L159 (-32.175, -11.13) -> (-27.675, -11.13)
  line L160 (-21.025, -11.13) -> (-21.025, -16.73)
  line L161 (-21.025, -16.73) -> (-25.525, -16.73)
  line L162 (-25.525, -16.73) -> (-25.525, -11.13)
  line L163 (-25.525, -11.13) -> (-21.025, -11.13)
  line L164 (-1.075, -11.13) -> (-1.075, -16.73)
  line L165 (-1.075, -16.73) -> (-5.575, -16.73)
  line L166 (-5.575, -16.73) -> (-5.575, -11.13)
  line L167 (-5.575, -11.13) -> (-1.075, -11.13)
  line L168 (-14.375, -11.13) -> (-14.375, -16.73)
  line L169 (-14.375, -16.73) -> (-18.875, -16.73)
  line L170 (-18.875, -16.73) -> (-18.875, -11.13)
  line L171 (-18.875, -11.13) -> (-14.375, -11.13)
  line L172 (-7.725, -11.13) -> (-7.725, -16.73)
  line L173 (-7.725, -16.73) -> (-12.225, -16.73)
  line L174 (-12.225, -16.73) -> (-12.225, -11.13)
  line L175 (-12.225, -11.13) -> (-7.725, -11.13)
  line L176 (5.575, -48.68) -> (5.575, -54.28)
  line L177 (5.575, -54.28) -> (1.075, -54.28)
  line L178 (1.075, -54.28) -> (1.075, -48.68)
  line L179 (1.075, -48.68) -> (5.575, -48.68)
  line L180 (-7.725, -48.68) -> (-7.725, -54.28)
  line L181 (-7.725, -54.28) -> (-12.225, -54.28)
  line L182 (-12.225, -54.28) -> (-12.225, -48.68)
  line L183 (-12.225, -48.68) -> (-7.725, -48.68)
  line L184 (-14.375, -48.68) -> (-14.375, -54.28)
  line L185 (-14.375, -54.28) -> (-18.875, -54.28)
  line L186 (-18.875, -54.28) -> (-18.875, -48.68)
  line L187 (-18.875, -48.68) -> (-14.375, -48.68)
  line L188 (-21.025, -48.68) -> (-21.025, -54.28)
  line L189 (-21.025, -54.28) -> (-25.525, -54.28)
  line L190 (-25.525, -54.28) -> (-25.525, -48.68)
  line L191 (-25.525, -48.68) -> (-21.025, -48.68)
  line L192 (-1.075, -48.68) -> (-1.075, -54.28)
  line L193 (-1.075, -54.28) -> (-5.575, -54.28)
  line L194 (-5.575, -54.28) -> (-5.575, -48.68)
  line L195 (-5.575, -48.68) -> (-1.075, -48.68)
  line L196 (-14.375, -41.17) -> (-14.375, -46.77)
  line L197 (-14.375, -46.77) -> (-18.875, -46.77)
  line L198 (-18.875, -46.77) -> (-18.875, -41.17)
  line L199 (-18.875, -41.17) -> (-14.375, -41.17)
  line L200 (-27.675, -48.68) -> (-27.675, -54.28)
  line L201 (-27.675, -54.28) -> (-32.175, -54.28)
  line L202 (-32.175, -54.28) -> (-32.175, -48.68)
  line L203 (-32.175, -48.68) -> (-27.675, -48.68)
  line L204 (10.1, 12.08) -> (-31.85, 12.08)
  line L205 (-31.85, 12.08) -> (-31.85, 56.38)
  line L206 (-31.85, 56.38) -> (31.85, 56.38)
  line L207 (31.85, 56.38) -> (31.85, 12.08)
  line L208 (31.85, 12.08) -> (14.6, 12.08)
  line L209 (14.6, 12.08) -> (14.6, 7.38)
  line L210 (14.6, 7.38) -> (10.1, 7.38)
  line L211 (10.1, 7.38) -> (10.1, 12.08)
  line L212 (12.225, -48.68) -> (12.225, -54.28)
  line L213 (12.225, -54.28) -> (7.725, -54.28)
  line L214 (7.725, -54.28) -> (7.725, -48.68)
  line L215 (7.725, -48.68) -> (12.225, -48.68)
  line L216 (18.875, -48.68) -> (18.875, -54.28)
  line L217 (18.875, -54.28) -> (14.375, -54.28)
  line L218 (14.375, -54.28) -> (14.375, -48.68)
  line L219 (14.375, -48.68) -> (18.875, -48.68)
  line L220 (25.525, -48.68) -> (25.525, -54.28)
  line L221 (25.525, -54.28) -> (21.025, -54.28)
  line L222 (21.025, -54.28) -> (21.025, -48.68)
  line L223 (21.025, -48.68) -> (25.525, -48.68)
  line L224 (32.175, -48.68) -> (32.175, -54.28)
  line L225 (32.175, -54.28) -> (27.675, -54.28)
  line L226 (27.675, -54.28) -> (27.675, -48.68)
  line L227 (27.675, -48.68) -> (32.175, -48.68)
  line L228 (-27.675, -41.17) -> (-27.675, -46.77)
  line L229 (-27.675, -46.77) -> (-32.175, -46.77)
  line L230 (-32.175, -46.77) -> (-32.175, -41.17)
  line L231 (-32.175, -41.17) -> (-27.675, -41.17)
  line L232 (-7.725, -41.17) -> (-7.725, -46.77)
  line L233 (-7.725, -46.77) -> (-12.225, -46.77)
  line L234 (-12.225, -46.77) -> (-12.225, -41.17)
  line L235 (-12.225, -41.17) -> (-7.725, -41.17)
  line L236 (-21.025, -41.17) -> (-21.025, -46.77)
  line L237 (-21.025, -46.77) -> (-25.525, -46.77)
  line L238 (-25.525, -46.77) -> (-25.525, -41.17)
  line L239 (-25.525, -41.17) -> (-21.025, -41.17)
  line L240 (-8.85, -3.12) -> (-13.35, -3.12)
  line L241 (-13.35, -3.12) -> (-13.35, 2.48)
  line L242 (-13.35, 2.48) -> (-8.85, 2.48)
  line L243 (-8.85, 2.48) -> (-8.85, -3.12)
  line L244 (-24.32, -3.12) -> (-28.82, -3.12)
  line L245 (-28.82, -3.12) -> (-28.82, 2.48)
  line L246 (-28.82, 2.48) -> (-24.32, 2.48)
  line L247 (-24.32, 2.48) -> (-24.32, -3.12)
  line L248 (-16.585, -8.15) -> (-21.085, -8.15)
  line L249 (-21.085, -8.15) -> (-21.085, -2.55)
  line L250 (-21.085, -2.55) -> (-16.585, -2.55)
  line L251 (-16.585, -2.55) -> (-16.585, -8.15)
  line L252 (16.585, -2.55) -> (21.085, -2.55)
  line L253 (21.085, -2.55) -> (21.085, -8.15)
  line L254 (21.085, -8.15) -> (16.585, -8.15)
  line L255 (16.585, -8.15) -> (16.585, -2.55)
  line L256 (-16.585, 7.51) -> (-16.585, 1.91)
  line L257 (-16.585, 1.91) -> (-21.085, 1.91)
  line L258 (-21.085, 1.91) -> (-21.085, 7.51)
  line L259 (-21.085, 7.51) -> (-16.585, 7.51)
  line L260 (16.585, 7.51) -> (21.085, 7.51)
  line L261 (21.085, 7.51) -> (21.085, 1.91)
  line L262 (21.085, 1.91) -> (16.585, 1.91)
  line L263 (16.585, 1.91) -> (16.585, 7.51)
  line L264 (24.32, 2.48) -> (28.82, 2.48)
  line L265 (28.82, 2.48) -> (28.82, -3.12)
  line L266 (28.82, -3.12) -> (24.32, -3.12)
  line L267 (24.32, -3.12) -> (24.32, 2.48)
  line L268 (8.85, 2.48) -> (13.35, 2.48)
  line L269 (13.35, 2.48) -> (13.35, -3.12)
  line L270 (13.35, -3.12) -> (8.85, -3.12)
  line L271 (8.85, -3.12) -> (8.85, 2.48)
  line L272 (32.175, -11.13) -> (32.175, -16.73)
  line L273 (32.175, -16.73) -> (27.675, -16.73)
  line L274 (27.675, -16.73) -> (27.675, -11.13)
  line L275 (27.675, -11.13) -> (32.175, -11.13)
  line L276 (25.525, -11.13) -> (25.525, -16.73)
  line L277 (25.525, -16.73) -> (21.025, -16.73)
  line L278 (21.025, -16.73) -> (21.025, -11.13)
  line L279 (21.025, -11.13) -> (25.525, -11.13)
  line L280 (18.875, -11.13) -> (18.875, -16.73)
  line L281 (18.875, -16.73) -> (14.375, -16.73)
  line L282 (14.375, -16.73) -> (14.375, -11.13)
  line L283 (14.375, -11.13) -> (18.875, -11.13)
  line L284 (12.225, -11.13) -> (12.225, -16.73)
  line L285 (12.225, -16.73) -> (7.725, -16.73)
  line L286 (7.725, -16.73) -> (7.725, -11.13)
  line L287 (7.725, -11.13) -> (12.225, -11.13)
  arc A4 (-34.05, 60.68) -> (-36.05, 58.68) centre (-34.05, 58.68) ccw
  line L288 (-36.05, 58.68) -> (-36.05, -58.68)
  arc A5 (-36.05, -58.68) -> (-34.05, -60.68) centre (-34.05, -58.68) ccw
  line L289 (-34.05, -60.68) -> (34.05, -60.68)
  arc A6 (34.05, -60.68) -> (36.05, -58.68) centre (34.05, -58.68) ccw
  line L290 (36.05, -58.68) -> (36.05, 58.68)
  arc A7 (36.05, 58.68) -> (34.05, 60.68) centre (34.05, 58.68) ccw
  line L291 (34.05, 60.68) -> (-34.05, 60.68)
  line L292 (18.875, -54.28) -> (14.375, -48.68) construction
  line L293 (-7.725, -54.28) -> (-12.225, -48.68) construction
  circle A8 centre (16.625, -51.48) radius 2.5
  circle A9 centre (-9.975, -51.48) radius 2.5
  line L294 (29.925, -11.13) -> (29.925, -7)
  line L295 (0, 29) -> (0, 6)
  circle A10 centre (29.925, -7) radius 2.5
  circle A11 centre (-29.925, -7) radius 2.5
  point P0 (-34.05, 58.68)
  point P1 (34.05, 58.68)
  point P2 (34.05, -58.68)
  point P3 (-34.05, -58.68)
  point P4 (-34.05, 58.68)
  point P5 (34.05, 58.68)
  point P6 (34.05, -58.68)
  point P7 (-34.05, -58.68)
  point P8 (-34.05, 58.68)
  point P9 (34.05, 58.68)
  point P10 (34.05, -58.68)
  point P11 (-34.05, -58.68)
  point P12 (-34.05, 58.68)
  point P13 (34.05, 58.68)
  point P14 (34.05, -58.68)
  point P15 (-34.05, -58.68)
  point P16 (-34.05, 58.68)
  point P17 (34.05, 58.68)
  point P18 (34.05, -58.68)
  point P19 (-34.05, -58.68)
  point P20 (-34.05, 58.68)
  point P21 (34.05, 58.68)
  point P22 (34.05, -58.68)
  point P23 (-34.05, -58.68)
  dimension "d145" = 5
  dimension "d146" = 5
  dimension "d149" = 5
  constraint coincident L216.end L217.start
  constraint coincident L218.end L219.start
  constraint coincident L180.end L181.start
  constraint coincident L182.end L183.start
  constraint midpoint L292 A8.centre
  constraint midpoint L293 A9.centre
  constraint midpoint L275 L294.start
  constraint perpendicular L275 L294
  constraint perpendicular L204 L295
  constraint coincident L294.end A10.centre
  constraint symmetric L295 A10 A11
  measures "d145" diameter of A8
  measures "d146" diameter of A9
  measures "d149" diameter of A10
extrude "Extrusion12" add sketch "Esquisse1" against normal blind 5.8 from surface at -4 contours L319 L322 L327 L328 L329 L330 L331 L332 | L319 L320 L333 L334 L335 L336 L337 L338 | L321 L322 L351 L352 L356 L358 | L320 L321 L359 L362 L364 L366 bodies 1
extrude "Extrusion14" add sketch "Esquisse3" along normal up to surface (12 mm away) separate body contours A0 L4 A1 L5 A2 L6 A3 L7 L288 L289 L290 L291 | A0 A4 | A1 A7 | A3 A5 | A2 A6 makes body 2
extrude "Extrusion15" cut sketch "Esquisse1" against normal blind 6 from surface at -4 contours L319 L322 L327 L328 L329 L330 L331 L332 | L319 L322 L329 L330 L331 L332 L345 L346 L347 L350 | L319 L320 L335 L336 L337 L338 L339 L340 L341 L344 | L321 L322 L351 L352 L353 L354 L355 L356 L357 L358 | L319 L320 L333 L334 L335 L336 L337 L338 | L321 L322 L351 L352 L356 L358 | L320 L321 L359 L360 L361 L362 L363 L364 L365 L366 | L320 L321 L359 L362 L364 L366 bodies 2